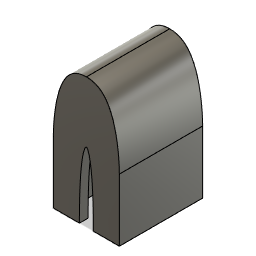
Zahnputz_Kappe (Autodesk Fusion 360 design; units mm, degrees)
Autodesk Fusion 360 part; units mm, degrees
note: some values were not read from the file. Set by a fixed rule: which sketch regions a step uses.
sketch "Skizze1" plane through (0, 0, 0) normal (0, 0, 1) x (1, 0, 0)
  line L0 (0, 0) -> (0, 35)
  line L1 (7, 0) -> (9.5, 0)
  line L2 (9.5, 0) -> (9.5, 18)
  line L3 (9.5, 18) -> (7, 18) construction
  line L4 (7, 18) -> (7, 0)
  spline S0 degree 5 poles (0, 35) (0.73, 35) (2.063, 34.7613) (3.6816, 33.688) (5.1796, 31.0566) (6.2948, 26.6703) (6.7786, 22.9675) (6.9597, 20.3756) (7, 18.7712) (7, 18) knots 0 0 0 0 0 0 0.2 0.4 0.6 0.8 1 1 1 1 1 1
  spline S1 degree 5 poles (0, 37.5) (0.9879, 37.5) (2.7924, 37.2385) (4.9853, 36.0627) (7.0185, 33.1717) (8.5367, 28.287) (9.1974, 24.0454) (9.445, 20.9552) (9.5, 18.9722) (9.5, 18) knots 0 0 0 0 0 0 0.2 0.4 0.6 0.8 1 1 1 1 1 1
  line L5 (0, 37.5) -> (0, 35)
  line L6 (-2.5, 37.5) -> (2.5, 37.5)
  line L7 (-1.5, 35) -> (1.5, 35)
  line L8 (7, 20) -> (7, 16)
  line L9 (9.5, 21) -> (9.5, 15)
  line L10 (0, 0) -> (7, 0)
  circle A0 centre (0, 16) radius 1
  line L11 (1, 16) -> (1, 0)
  line L12 (0, 0) -> (0, -5) construction
  line L13 (0, 37.5) -> (0, 35)
  line L14 (-1, 16) -> (-1, 0)
  line L15 (-7, 20) -> (-7, 16)
  circle A1 centre (0, 16) radius 1
  spline S2 degree 5 poles (0, 37.5) (-0.9879, 37.5) (-2.7924, 37.2385) (-4.9853, 36.0627) (-7.0185, 33.1717) (-8.5367, 28.287) (-9.1974, 24.0454) (-9.445, 20.9552) (-9.5, 18.9722) (-9.5, 18) knots 0 0 0 0 0 0 0.2 0.4 0.6 0.8 1 1 1 1 1 1
  line L16 (2.5, 37.5) -> (-2.5, 37.5)
  line L17 (-9.5, 21) -> (-9.5, 15)
  line L18 (-9.5, 21) -> (-9.5, 15)
  line L19 (0, 0) -> (-7, 0)
  line L20 (-9.5, 0) -> (-9.5, 18)
  line L21 (-9.5, 18) -> (-7, 18) construction
  spline S3 degree 5 poles (0, 35) (-0.73, 35) (-2.063, 34.7613) (-3.6816, 33.688) (-5.1796, 31.0566) (-6.2948, 26.6703) (-6.7786, 22.9675) (-6.9597, 20.3756) (-7, 18.7712) (-7, 18) knots 0 0 0 0 0 0 0.2 0.4 0.6 0.8 1 1 1 1 1 1
  line L22 (1.5, 35) -> (-1.5, 35)
  line L23 (-7, 20) -> (-7, 16)
  line L24 (-7, 0) -> (-9.5, 0)
  line L25 (-7, 18) -> (-7, 0)
  line L26 (0, 0) -> (0, 35)
  line L27 (1.5, 35) -> (-1.5, 35)
  line L28 (2.5, 37.5) -> (-2.5, 37.5)
  dimension "d1" = 18
  dimension "d2" = 5
  dimension "d3" = 3
  dimension "d4" = 4
  dimension "d5" = 6
  dimension "d6" = 7
  dimension "d7" = 35
  dimension "d8" = 2.5
  dimension "d9" = 16
  dimension "d10" = 2
  constraint coincident L0.start L10.start
  constraint vertical L0
  constraint horizontal L1
  constraint vertical L2
  constraint horizontal L3
  constraint vertical L4
  constraint parallel L0 L5
  constraint equal L1 L5
  constraint midpoint S1.start L6
  constraint perpendicular L5 L6
  constraint midpoint L0.end L7
  constraint perpendicular L0 L7
  constraint midpoint L3.end L8
  constraint midpoint L2.end L9
  constraint perpendicular L4 L10
  constraint coincident L0 A0.centre
  constraint coincident A0 L11.start
  constraint coincident L10 L11.end
  constraint tangent A0 L11
  constraint perpendicular L10 L11
  constraint perpendicular L10 L12
  constraint symmetric L0.start L12 L10.start
  constraint symmetric L0.end L12 S0.start
  constraint symmetric L1.start L12 L19.end
  constraint symmetric L1.end L12 L20.start
  constraint symmetric L2.end L12 S2.end
  constraint symmetric L3.end L12 L21.end
  constraint symmetric S1.start L12 L5.start
  constraint symmetric L6.start L12 L6.end
  constraint symmetric L6.end L12 L6.start
  constraint symmetric L7.start L12 L7.end
  constraint symmetric L7.end L12 L7.start
  constraint symmetric L8.start L12 L15.start
  constraint symmetric L8.end L12 L15.end
  constraint symmetric L9.start L12 L17.start
  constraint symmetric L9.end L12 L17.end
  constraint symmetric A0 L12 A1
  constraint symmetric L11.start L12 L14.start
  constraint symmetric L11.end L12 L14.end
  measures "d1" distance of L1.end L2.end
  measures "d2" distance of L6.start L6.end
  measures "d3" distance of L7.start L7.end
  measures "d4" distance of L8.start L8.end
  measures "d5" distance of L9.start L9.end
  measures "d6" distance of L0 L4
  measures "d7" distance of L0.start L0.end
  measures "d8" distance of L1.start L1.end
  measures "d9" distance of L10 A0.centre
  measures "d10" diameter of A0
extrude "Extrusion1" add sketch "Skizze1" along normal mid plane 24
shell "Schale1" thickness 2.5 removed faces 1 at (3.1667, 0, 4)
sketch "Skizze2" plane through (0, 0, 12) normal (0, 0, 1) x (1, 0, 0)
  line L0 (-9.5, 0) -> (9.5, 0)
  line L1 (9.5, 0) -> (9.5, 18)
  spline S0 degree 5 poles (9.5, 18) (9.5, 18.9722) (9.445, 20.9552) (9.1974, 24.0454) (8.5367, 28.287) (7.0185, 33.1717) (4.9853, 36.0627) (2.7924, 37.2385) (0.9879, 37.5) (0, 37.5) knots -1 -1 -1 -1 -1 -1 -0.8 -0.6 -0.4 -0.2 0 0 0 0 0 0
  spline S1 degree 5 poles (0, 37.5) (-0.9879, 37.5) (-2.7924, 37.2385) (-4.9853, 36.0627) (-7.0185, 33.1717) (-8.5367, 28.287) (-9.1974, 24.0454) (-9.445, 20.9552) (-9.5, 18.9722) (-9.5, 18) knots 0 0 0 0 0 0 0.2 0.4 0.6 0.8 1 1 1 1 1 1
  line L2 (-9.5, 18) -> (-9.5, 0)
  spline S2 degree 5 poles (-2, 0) (-2, 2.2036) (-1.9635, 6.2369) (-1.7993, 11.1651) (-1.4009, 15.6523) (-0.8096, 18.6119) (-0.3036, 19.8562) (-0.0021, 20.1554) (0.2998, 19.8561) (0.8069, 18.6119) (1.3996, 15.6524) (1.7989, 11.1652) (1.9634, 6.237) (2, 2.2037) (2, 0) knots 0 0 0 0 0 0 0.1 0.2 0.3 0.4 0.5 0.6 0.7 0.8 0.9 1 1 1 1 1 1
  line L3 (0, 0) -> (-0.002, 20) construction
  line L4 (-0.102, 20) -> (0.098, 20)
  line L5 (2, 5) -> (2, -5)
  line L6 (-2, -5) -> (-2, 5)
  point P0 (-0.002, 20)
  dimension "d14" = 4
  dimension "d15" = 10
  dimension "d16" = 0.2
  dimension "d17" = 20
  constraint coincident L0 S2.start
  constraint coincident L0 S2.end
  constraint coincident L3.start origin
  constraint coincident P0 L3.end
  constraint midpoint P0 L4
  constraint horizontal L4
  constraint midpoint S2.end L5
  constraint vertical L5
  constraint midpoint S2.start L6
  constraint vertical L6
  constraint equal L5 L6
  measures "d14" distance of L5 L6
  measures "d15" distance of L5.start L5.end
  measures "d16" distance of L4.start L4.end
  measures "d17" vertical distance of L3.start P0
extrude "Extrusion2" cut sketch "Skizze2" against normal blind 24 contours L0 S2
